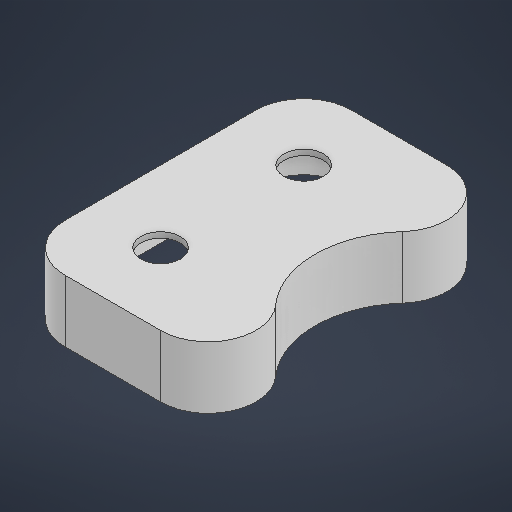
# Autodesk Inventor part: ControllerTop
Saved by Autodesk Inventor 2026.1 (Build 301233000, 233)
## iProperties
Created: 2026-07-05
Part Number: ControllerTop
Material: Generic
Document SubType Name: Modeling
Designer: Kasi Pusuluri
Density: 1 g/cm^3
Appearance: Default
Author: Kasi Pusuluri
Autodesk Inventor part; units mm, degrees
ref_plane "YZ Plane" through (0, 0, 0) normal (1, 0, 0) x (0, 1, 0)
ref_plane "XZ Plane" through (0, 0, 0) normal (0, 1, 0) x (-1, 0, 0)
ref_plane "XY Plane" through (0, 0, 0) normal (0, 0, 1) x (1, 0, 0)
sketch "Sketch1" plane through (0, 0, 0) normal (0, 1, 0) x (-1, 0, 0)
  line L0 (-25.4, 76.2) -> (25.4, 76.2)
  line L1 (50.8, 76.2) -> (-50.8, 76.2)
  line L2 (-50.8, 50.8) -> (-50.8, -50.8)
  line L3 (50.8, 76.2) -> (-50.8, 76.2)
  line L4 (-25.4, -76.2) -> (25.4, -76.2)
  line L5 (50.8, -50.8) -> (50.8, 50.8)
  arc A0 (50.8, 50.8) -> (25.4, 76.2) centre (25.4, 50.8) ccw
  arc A1 (25.4, -76.2) -> (50.8, -50.8) centre (25.4, -50.8) ccw
  arc A2 (-50.8, -50.8) -> (-25.4, -76.2) centre (-25.4, -50.8) ccw
  arc A3 (-25.4, 76.2) -> (-50.8, 50.8) centre (-25.4, 50.8) ccw
  circle A4 centre (-25.4, 50.8) radius 25.4
  circle A5 centre (-25.4, -50.8) radius 25.4
  circle A6 centre (-50.8, 0) radius 31.3961
  circle A7 centre (-82.1961, 0) radius 50.8
  circle A8 centre (25.4, -50.8) radius 2.5
  circle A9 centre (25.4, -50.8) radius 1.25
  circle A10 centre (25.4, 50.8) radius 2.5
  circle A11 centre (25.4, 50.8) radius 1.25
  circle A12 centre (-25.4, 50.8) radius 2.5
  circle A13 centre (-25.4, 50.8) radius 1.25
  circle A14 centre (-25.4, -50.8) radius 2.5
  circle A15 centre (-25.4, -50.8) radius 1.25
  line L6 (-31.3961, 0) -> (50.8, 0)
  point P0 (-36.7592, 28.0815)
  point P1 (-36.7592, -28.0815)
  point P2 (12.7, 38.1)
  point P3 (12.7, -38.1)
  point P4 (-50.8, -31.3961)
  point P5 (-50.8, 31.3961)
  point P6 (-44.332, -33.8667)
  point P7 (-44.332, 33.8667)
  point P8 (9.7019, 0)
  point P9 (0.3879, -59.1619)
  point P10 (-13.7063, -28.2519)
  dimension "d6" = 101.6
  dimension "d21" = 25.4
  dimension "d68" = 2.5
  dimension "d69" = 2.5
  dimension "d70" = 2.5
  dimension "d71" = 2.5
  dimension "d72" = 5
  dimension "d73" = 5
  dimension "d74" = 5
  dimension "d75" = 5
  constraints: 14 end point, 13 centre point, 10 coincident, 8 point on circle, 8 tangent, 4 equal radius, 4 point on line, 3 horizontal, 2 midpoint, 1 parallel, 1 perpendicular, 11 other
  measures "d6" distance of point (-50.8, 76.2) L1.start
  measures "d21" radius of A0
  measures "d68" diameter of A9
  measures "d69" diameter of A11
  measures "d70" diameter of A13
  measures "d71" diameter of A15
  measures "d72" diameter of A8
  measures "d73" diameter of A10
  measures "d74" diameter of A12
  measures "d75" diameter of A14
extrude "Extrusion4" add sketch "Sketch1" along normal blind 3 contours A4 A3 | L0 A0 L5 L6 A6 A4 | A4 A6 A7 | A6 L6 A7 | L5 A1 L4 A5 A6 L6 | A6 A7 L6 | A5 A2 | A7 A6 A5 | A8 | A9 | A10 | A11 | A12 | A13 | A14 | A15
hole "Hole3" at (-12.7, 0, 38.1) at (-12.7, 0, -38.1) direction (0, 1, 0) diameter 21 depth 25.4 tip angle 118
sketch "Sketch5" plane through (0, 0, 0) normal (0, -1, 0) x (1, 0, 0)
  arc A0 (36.7592, 28.0815) -> (36.7592, -28.0815) centre (50.8, 0) ccw projected
  arc A1 (36.7592, 28.0815) -> (36.7592, -28.0815) centre (50.8, 0) ccw
  arc A2 (44.332, 33.8667) -> (25.4, 76.2) centre (25.4, 50.8) ccw projected
  arc A3 (36.7592, 28.0815) -> (25.4, 76.2) centre (25.4, 50.8) ccw
  arc A4 (25.4, -76.2) -> (44.332, -33.8667) centre (25.4, -50.8) ccw projected
  arc A5 (25.4, -76.2) -> (36.7592, -28.0815) centre (25.4, -50.8) ccw
  arc A6 (-25.4, 76.2) -> (-50.8, 50.8) centre (-25.4, 50.8) ccw projected
  line L0 (-50.8, -50.8) -> (-50.8, 50.8) projected
  arc A7 (-25.4, 76.2) -> (-50.8, 50.8) centre (-25.4, 50.8) ccw
  arc A8 (-50.8, -50.8) -> (-25.4, -76.2) centre (-25.4, -50.8) ccw projected
  arc A9 (-50.8, -50.8) -> (-25.4, -76.2) centre (-25.4, -50.8) ccw
  line L1 (-25.4, 76.2) -> (25.4, 76.2) projected
  line L2 (25.4, 76.2) -> (-25.4, 76.2)
  line L3 (25.4, -76.2) -> (-25.4, -76.2) projected
  line L4 (25.4, -76.2) -> (-25.4, -76.2)
  line L5 (-50.8, 50.8) -> (-50.8, -50.8)
  arc A10 (44.332, 33.8667) -> (25.4, 76.2) centre (25.4, 50.8) ccw
  arc A11 (44.332, 33.8667) -> (44.332, -33.8667) centre (82.1961, 0) ccw projected
  arc A12 (44.332, 33.8667) -> (44.332, -33.8667) centre (82.1961, 0) ccw
  arc A13 (25.4, -76.2) -> (44.332, -33.8667) centre (25.4, -50.8) ccw
  arc A14 (-50.8, -50.8) -> (-25.4, -76.2) centre (-25.4, -50.8) ccw
  arc A15 (-25.4, 76.2) -> (-50.8, 50.8) centre (-25.4, 50.8) ccw projected
  arc A16 (-25.4, 76.2) -> (-50.8, 50.8) centre (-25.4, 50.8) ccw
  line L6 (-25.4, 76.2) -> (25.4, 76.2)
  line L7 (-50.8, 50.8) -> (-50.8, -50.8)
  line L8 (-25.4, -76.2) -> (25.4, -76.2)
  point P0 (0, 0)
  point P1 (-12.7, 38.1)
  point P2 (-12.7, -38.1)
  constraints: 22 point on circle, 12 end point, 11 tangent, 10 centre point, 3 horizontal, 2 perpendicular, 1 concentric, 1 vertical
extrude "Extrusion5" add sketch "Sketch5" along normal blind 30
shell "Shell1" thickness 3 removed faces 3 at (-23.4013, -30, 0) at (-13.5376, 0, 41.4983) at (-15.9531, 0, -34.6)
sketch "Sketch8" plane through (-50.8, 3, -50.8) normal (-1, 0, 0) x (0, 0, 1)
  line L0 (0, -33) -> (101.6, -33) projected
  line L1 (0, 0) -> (101.6, 0)
  line L2 (101.6, 0) -> (101.6, -33)
  line L3 (101.6, -33) -> (0, -33)
  line L4 (0, -33) -> (0, 0)
  line L5 (50.8, 0) -> (50.8, -33)
  line L6 (0, -16.5) -> (101.6, -16.5)
  line L7 (50.8, -16.5) -> (55.1, -16.5)
  line L8 (55.1, -16.5) -> (55.1, -14.7)
  line L9 (50.8, -16.5) -> (46.5, -16.5)
  line L10 (46.5, -16.5) -> (46.5, -18.3)
  line L11 (55.1, -14.7) -> (46.5, -14.7)
  line L12 (46.5, -14.7) -> (46.5, -18.3)
  line L13 (46.5, -18.3) -> (55.1, -18.3)
  line L14 (55.1, -18.3) -> (55.1, -14.7)
  point P0 (50.8, -3)
  dimension "d82" = 4.3
  dimension "d83" = 4.3
  dimension "d84" = 1.8
  dimension "d85" = 1.8
  constraints: 28 end point, 6 midpoint, 4 parallel, 2 horizontal, 2 perpendicular, 2 point on line, 2 vertical
  measures "d82" distance of L7.end point (50.8, -16.5)
  measures "d83" distance of L9.end L7.start
  measures "d84" distance of L9.end L10.end
  measures "d85" distance of L7.end L8.end
extrude "Extrusion8" cut sketch "Sketch8" against normal blind 2.54 contours L13 L10 L6 L5 | L5 L6 L14 L13 | L12 L11 L5 L6 | L5 L11 L8 L6
extrude "Extrusion9" add sketch "Sketch1" against normal blind 3 contours A8 | A10 | A12 | A14
equation "\"d69\" = d68"
equation "\"d70\" = d68"
equation "\"d71\" = d68"
equation "\"d73\" = d72"
equation "\"d74\" = d73"
equation "\"d75\" = d72"
equation "\"d83\" = d82"
equation "\"d85\" = d84"
body "Solid3"
